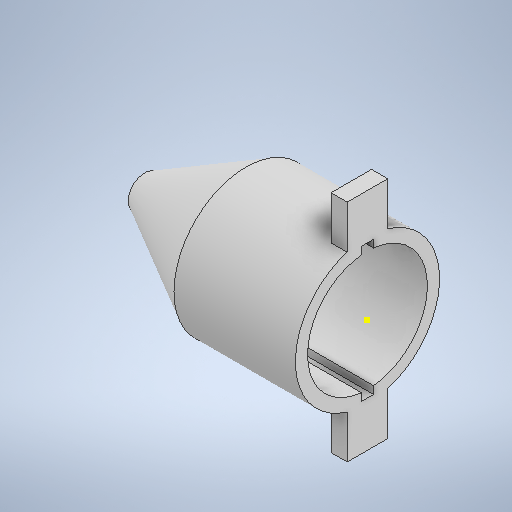
# Autodesk Inventor part: Joy stick part 2
Saved by Autodesk Inventor 2025.2 (Build 292293000, 293)
## iProperties
Created: 2025-04-03
Part Number: Joy stick part 2
Material: Generic
Document SubType Name: Modeling
Designer: avnr2
Density: 1 g/cm^3
Appearance: Default
Author: avnr2
Autodesk Inventor part; units mm, degrees
ref_plane "YZ Plane" through (0, 0, 0) normal (1, 0, 0) x (0, 1, 0)
ref_plane "XZ Plane" through (0, 0, 0) normal (0, 1, 0) x (-1, 0, 0)
ref_plane "XY Plane" through (0, 0, 0) normal (0, 0, 1) x (1, 0, 0)
sketch "Sketch1" plane through (0, 0, 0) normal (0, 1, 0) x (-1, 0, 0)
  line L0 (0, 0) -> (12.5354, 0)
  line L1 (12.5354, 0) -> (12.5354, -2)
  line L2 (12.5354, -2) -> (0, -8.897)
  line L3 (0, -8.897) -> (0, -7.397)
  line L4 (10.9043, 0) -> (10.9043, -1.3974)
  line L5 (0, -7.397) -> (10.9043, -1.3974)
  dimension "d0" = 2
  dimension "d23" = 1.5
  constraints: 12 end point, 3 vertical, 1 horizontal, 1 parallel, 1 point on line, 1 vertical alignment
  measures "d0" distance of L0.end L1.end
  measures "d23" distance of L2.end L3.end
revolve "Revolution1" add sketch "Sketch1" angle 360 about axis through (0, 0, 0) along (-1, 0, 0)
sketch "Sketch2" plane through (0, 0, 0) normal (1, 0, 0) x (0, 0, -1)
  point P0 (0, 0)
sketch "Sketch3" plane through (-12.5354, 0, 0) normal (-1, 0, 0) x (0, 0, 1)
  point P0 (0, 0)
sketch "Sketch4" plane through (-12.5354, 0, 0) normal (-1, 0, 0) x (0, 0, 1)
  circle A0 centre (0, 0) radius 1.5
  dimension "d37" = 3
  constraints: 1 centre point, 1 coincident
  measures "d37" diameter of A0
sketch "Sketch5" plane through (-12.5354, 0, 0) normal (-1, 0, 0) x (0, 0, 1)
  point P0 (0, 0)
extrude "Extrusion1" cut sketch "Sketch4" against normal blind 10
sketch "Sketch6" plane through (-2.3704, 0, 0) normal (-1, 0, 0) x (0, 0, 1)
  circle A0 centre (0, 0) radius 2
  constraints: 1 centre point, 1 coincident
sketch "Sketch7" plane through (0, 0, 0) normal (1, 0, 0) x (0, 0, -1)
  circle A0 centre (0, 0) radius 8.897
  constraints: 1 centre point, 1 coincident
extrude "Extrusion2" [suppressed]
sketch "Sketch8" plane through (15, 0, 0) normal (1, 0, 0) x (0, 0, -1)
  circle A0 centre (0, 0) radius 8.897 projected
  line L0 (-8.6693, -2) -> (-13.1693, -2)
  line L1 (-13.1693, -2) -> (-13.1693, 0)
  line L2 (-13.1693, 0) -> (-8.897, 0)
  line L3 (-8.6693, 2) -> (-13.1693, 2)
  line L4 (-13.1693, 2) -> (-13.1693, 0)
  line L5 (0, -8.897) -> (0, 8.897)
  line L6 (8.6693, -2) -> (13.1693, -2)
  line L7 (13.1693, -2) -> (13.1693, 0)
  line L8 (13.1693, 0) -> (8.897, 0)
  line L9 (8.6693, 2) -> (13.1693, 2)
  line L10 (13.1693, 2) -> (13.1693, 0)
  dimension "d8" = 4.5
  dimension "d9" = 2
  constraints: 22 end point, 8 symmetric about line, 4 point on circle, 2 perpendicular, 1 horizontal, 1 horizontal alignment, 1 vertical
  measures "d8" distance of L0.start L0.end
  measures "d9" distance of L0.end L1.end
extrude "Extrusion3" [suppressed]
sketch "Sketch9" plane through (15, 0, 0) normal (1, 0, 0) x (0, 0, -1)
  point P0 (0, 0)
sketch "Sketch10" plane through (15, 0, 0) normal (1, 0, 0) x (0, 0, -1)
  point P0 (0, 0)
sketch "Sketch11" plane through (15, 0, 0) normal (1, 0, 0) x (0, 0, -1)
  point P0 (0, 0)
sketch "Sketch12" plane through (15, 0, 0) normal (1, 0, 0) x (0, 0, -1)
  circle A0 centre (0, 0) radius 7.5
  dimension "d12" = 15
  constraints: 1 centre point, 1 coincident
  measures "d12" diameter of A0
sketch "Sketch13" plane through (15, 0, 0) normal (1, 0, 0) x (0, 0, -1)
  line L0 (6.4465, 0.75) -> (8.4465, 0.75)
  line L1 (8.4465, 0.75) -> (8.4465, -0.75)
  line L2 (8.4465, -0.75) -> (6.4465, -0.75)
  line L3 (6.4465, -0.75) -> (6.4465, 0.75)
  line L4 (6.4465, 0.75) -> (8.4465, -0.75) construction
  line L5 (8.4465, 0.75) -> (6.4465, -0.75) construction
  line L6 (0, 7.445) -> (0, -3.9697)
  line L7 (-6.4465, 0.75) -> (-8.4465, 0.75)
  line L8 (-8.4465, 0.75) -> (-8.4465, -0.75)
  line L9 (-8.4465, -0.75) -> (-6.4465, -0.75)
  line L10 (-6.4465, -0.75) -> (-6.4465, 0.75)
  line L11 (-6.4465, 0.75) -> (-8.4465, -0.75) construction
  line L12 (-8.4465, 0.75) -> (-6.4465, -0.75) construction
  point P0 (0, 0)
  point P1 (7.4465, 0)
  point P2 (-7.4465, 0)
  dimension "d13" = 2
  dimension "d14" = 1.5
  constraints: 26 end point, 5 symmetric about line, 2 midpoint, 2 parallel, 1 horizontal, 1 horizontal alignment, 1 perpendicular, 1 vertical
  measures "d13" distance of L1.end L2.end
  measures "d14" distance of L0.end L1.end
extrude "Extrusion4" [suppressed]
extrude "Extrusion5" [suppressed]
extrude "Extrusion6" [suppressed]
sketch "Sketch14" plane through (-2.3704, 0, 0) normal (-1, 0, 0) x (0, 0, 1)
  circle A0 centre (0, 0) radius 2
  constraints: 1 centre point, 1 coincident
extrude "Extrusion7" [suppressed]
sketch "Sketch15" plane through (0, 0, 0) normal (1, 0, 0) x (0, 0, -1)
  circle A0 centre (0, 0) radius 8.897
  circle A1 centre (0, 0) radius 7.397
  constraints: 2 centre point, 2 coincident
extrude "Extrusion8" add sketch "Sketch15" along normal blind 15
sketch "Sketch16" plane through (15, 0, 0) normal (1, 0, 0) x (0, 0, -1)
  point P0 (0, 0)
sketch "Sketch17" plane through (15, 0, 0) normal (1, 0, 0) x (0, 0, -1)
  circle A0 centre (0, 0) radius 8.897 projected
  line L0 (0, 8.897) -> (0, 13.897)
  line L1 (0, 13.897) -> (-2.5, 13.897)
  line L2 (-2.5, 13.897) -> (-2.5, 8.5385)
  line L3 (0, 13.897) -> (2.5, 13.897)
  line L4 (2.5, 13.897) -> (2.5, 8.5385)
  line L5 (-7.2862, 0) -> (2, 0)
  circle A1 centre (0, 0) radius 2 projected
  line L6 (0, -8.897) -> (0, -13.897)
  line L7 (0, -13.897) -> (-2.5, -13.897)
  line L8 (-2.5, -13.897) -> (-2.5, -8.5385)
  line L9 (0, -13.897) -> (2.5, -13.897)
  line L10 (2.5, -13.897) -> (2.5, -8.5385)
  dimension "d29" = 5
  dimension "d30" = 2.5
  constraints: 22 end point, 8 symmetric about line, 2 perpendicular, 2 point on circle, 1 horizontal, 1 horizontal alignment, 1 vertical, 1 other
  measures "d29" distance of L0.start L0.end
  measures "d30" distance of L0.end L1.end
extrude "Extrusion9" add sketch "Sketch17" against normal blind 2 contours A0 L0 L3 L4 | L10 L9 L6 A0 | A0 L2 L1 L0 | L6 L7 L8 A0
sketch "Sketch18" plane through (15, 0, 0) normal (1, 0, 0) x (0, 0, -1)
  circle A0 centre (0, 0) radius 7.397 projected
  line L0 (0, -7.397) -> (0, -8.297)
  line L1 (0, -8.297) -> (-0.75, -8.297)
  line L2 (-0.75, -8.297) -> (-0.75, -7.3588)
  line L3 (0, -8.297) -> (0.75, -8.297)
  line L4 (0.75, -8.297) -> (0.75, -7.3588)
  line L5 (-4.4895, 0) -> (3.1188, 0)
  line L6 (0, 7.397) -> (0, 8.297)
  line L7 (0, 8.297) -> (-0.75, 8.297)
  line L8 (-0.75, 8.297) -> (-0.75, 7.3588)
  line L9 (0, 8.297) -> (0.75, 8.297)
  line L10 (0.75, 8.297) -> (0.75, 7.3588)
  dimension "d33" = 0.9
  dimension "d34" = 0.75
  constraints: 22 end point, 8 symmetric about line, 2 point on circle, 2 vertical, 1 horizontal, 1 perpendicular
  measures "d33" distance of L0.start L0.end
  measures "d34" distance of L0.end L1.end
extrude "Extrusion10" cut sketch "Sketch18" against normal blind 10 contours A0 L6 L9 L10 | L4 L3 L0 A0 | A0 L8 L7 L6 | L0 L1 L2 A0
sketch "Sketch19" plane through (15, 0, 0) normal (1, 0, 0) x (0, 0, -1)
  point P0 (0, 0)
thread "Thread3" size "M3x0.5" class "6H" standard "ANSI Metric M Profile" length 10
body "Solid1"
